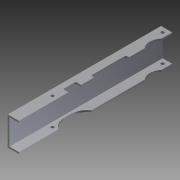
# Autodesk Inventor part: 2.25 U frame
Saved by Autodesk Inventor 2012 (Build 160160000, 160)
## iProperties
Created: 2013-11-04
Part Number: 2.25 U frame
Material: Default
Document SubType Name: Modeling
Designer: Bryce
Density: 1 g/cm^3
Author: Bryce
Autodesk Inventor part; units mm, degrees
ref_plane "YZ Plane" through (0, 0, 0) normal (1, 0, 0) x (0, 1, 0)
ref_plane "XZ Plane" through (0, 0, 0) normal (0, 1, 0) x (-1, 0, 0)
ref_plane "XY Plane" through (0, 0, 0) normal (0, 0, 1) x (1, 0, 0)
sketch "Sketch1" plane through (0, 0, 0) normal (0, 0, 1) x (1, 0, 0)
  line L0 (0, 0) -> (22.225, 0)
  line L1 (22.225, 0) -> (22.225, 57.15)
  line L2 (22.225, 57.15) -> (0, 57.15)
  line L3 (0, 57.15) -> (0, 0)
  line L4 (3.175, 3.175) -> (22.225, 3.175)
  line L5 (22.225, 3.175) -> (22.225, 53.975)
  line L6 (22.225, 53.975) -> (3.175, 53.975)
  line L7 (3.175, 53.975) -> (3.175, 3.175)
  dimension "d0" = 3.175
  dimension "d1" = 3.175
  dimension "d2" = 3.175
  dimension "d3" = 57.15
  dimension "d4" = 22.225
  constraints: 16 end point, 4 parallel, 2 horizontal, 2 perpendicular, 1 point on line
  measures "d0" distance between parallel lines of L0 L4
  measures "d1" distance between parallel lines of L3 L7
  measures "d2" distance between parallel lines of L6 L2
  measures "d3" distance of L2.end L0.start
  measures "d4" distance of L0.start L0.end
extrude "Extrusion1" add sketch "Sketch1" along normal blind 304.8 contours L3 L2 L1 L6 L7 L4 L0
sketch "Sketch2" plane through (0, 57.15, 0) normal (0, 1, 0) x (1, 0, 0)
  line L0 (22.225, 0) -> (22.225, -304.8) projected
  line L1 (22.225, 0) -> (0, 0) projected
  line L2 (22.225, -85.725) -> (15.875, -85.725)
  line L3 (15.875, -85.725) -> (15.875, -155.575)
  line L4 (15.875, -155.575) -> (22.225, -155.575)
  line L5 (22.225, -155.575) -> (22.225, -85.725)
  line L6 (0, 0) -> (0, -304.8) projected
  line L7 (22.225, -180.975) -> (11.43, -180.975)
  line L8 (11.43, -180.975) -> (11.43, -206.375)
  line L9 (11.43, -206.375) -> (22.225, -206.375)
  line L10 (22.225, -206.375) -> (22.225, -180.975)
  arc A0 (22.225, -21.2995) -> (22.225, -54.9005) centre (41.275, -38.1) ccw
  circle A1 centre (12.7, -9.525) radius 3.175
  circle A2 centre (12.7, -228.6) radius 3.175
  dimension "d11" = 85.725
  dimension "d12" = 69.85
  dimension "d13" = 6.35
  dimension "d14" = 180.975
  dimension "d15" = 25.4
  dimension "d16" = 11.43
  dimension "d24" = 25.4
  dimension "d25" = 41.275
  dimension "d26" = 38.1
  dimension "d27" = 12.7
  dimension "d28" = 9.525
  dimension "d29" = 6.35
  dimension "d30" = 228.6
  constraints: 16 end point, 4 parallel, 4 point on line, 3 centre point, 2 horizontal, 2 perpendicular, 2 point on circle, 1 equal radius, 1 vertical alignment
  measures "d11" distance between parallel lines of L1 L2
  measures "d12" distance of L2.end L3.end
  measures "d13" distance of L2.start L2.end
  measures "d14" distance between parallel lines of L1 L7
  measures "d15" distance between parallel lines of L9 L7
  measures "d16" distance between parallel lines of L6 L8
  measures "d24" radius of A0
  measures "d25" distance from line of A0.centre L6
  measures "d26" distance from line of A0.centre L1
  measures "d27" distance from line of A1.centre L6
  measures "d28" distance from line of L1 A1.centre
  measures "d29" diameter of A1
  measures "d30" distance from line of L1 A2.centre
extrude "Extrusion2" cut sketch "Sketch2" against normal blind 3.175
sketch "Sketch3" plane through (0, 0, 0) normal (0, -1, 0) x (1, 0, 0)
  line L0 (0, 0) -> (0, 304.8) projected
  line L1 (0, 0) -> (22.225, 0) projected
  line L2 (22.225, 0) -> (22.225, 304.8) projected
  arc A0 (7.9375, 187.325) -> (22.225, 160.8085) centre (39.6875, 187.325) ccw
  line L3 (7.9375, 187.325) -> (7.9375, 200.025)
  arc A1 (22.225, 226.5415) -> (7.9375, 200.025) centre (39.6875, 200.025) ccw
  arc A2 (22.225, 54.9005) -> (22.225, 21.2995) centre (41.275, 38.1) ccw projected
  circle A3 centre (12.7, 9.525) radius 3.175 projected
  circle A4 centre (12.7, 228.6) radius 3.175 projected
  dimension "d17" = 31.75
  dimension "d18" = 12.7
  dimension "d19" = 187.325
  dimension "d20" = 7.9375
  constraints: 4 point on circle, 2 centre point, 2 end point, 2 point on line, 2 tangent, 1 equal radius
  measures "d17" radius of A0
  measures "d18" distance of L3.start L3.end
  measures "d19" distance from line of L1 L3.start
  measures "d20" distance between parallel lines of L3 L0
extrude "Extrusion3" cut sketch "Sketch3" against normal blind 3.175
fillet "Fillet1" radius 3.175 4 edges at (15.875, 55.5625, 85.725) (15.875, 55.5625, 155.575) (11.43, 55.5625, 180.975) (11.43, 55.5625, 206.375)
equation "\"d1\" = d0"
equation "\"d2\" = d0"
body "Solid1"
